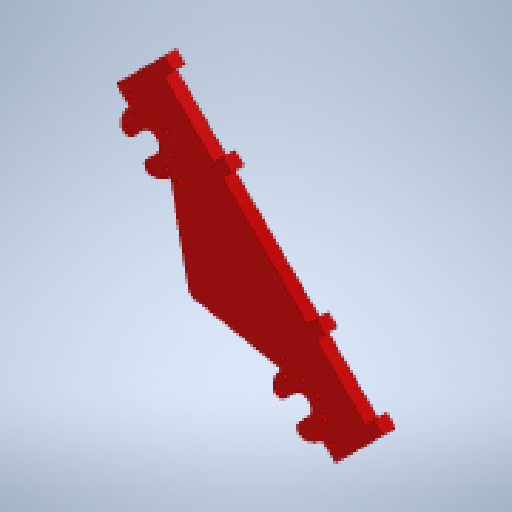
# Autodesk Inventor part: new_waist
Saved by Autodesk Inventor 2024 (Build 280153000, 153)
## iProperties
Created: 2024-09-05
Part Number: new_waist
Material: PMMA 플라스틱
Document SubType Name: Modeling
Designer: Eungang
Density: 1.188 g/cm^3
Appearance: 빨간색
Author: Eungang
Autodesk Inventor part; units mm, degrees
ref_plane "YZ Plane" through (0, 0, 0) normal (1, 0, 0) x (0, 1, 0)
ref_plane "XZ Plane" through (0, 0, 0) normal (0, 1, 0) x (-1, 0, 0)
ref_plane "XY Plane" through (0, 0, 0) normal (0, 0, 1) x (1, 0, 0)
sketch "스케치1" plane through (0, 0, 0) normal (0, 0, 1) x (1, 0, 0)
  circle A0 centre (0, 0) radius 13.8
  circle A1 centre (0, 0) radius 7.2
  circle A2 centre (0, 11) radius 1.28125
  circle A3 centre (-7.778175, 7.778175) radius 1.28125
  circle A4 centre (-11, 0) radius 1.28125
  circle A5 centre (-7.778175, -7.778175) radius 1.28125
  circle A6 centre (0, -11) radius 1.28125
  circle A7 centre (7.778175, -7.778175) radius 1.28125
  circle A8 centre (11, 0) radius 1.28125
  circle A9 centre (7.778175, 7.778175) radius 1.28125
  circle A10 centre (-7.778175, 7.778175) radius 1.025
  circle A11 centre (0, 11) radius 1.025
  circle A12 centre (7.778175, 7.778175) radius 1.025
  circle A13 centre (11, 0) radius 1.025
  circle A14 centre (7.778175, -7.778175) radius 1.025
  circle A15 centre (0, -11) radius 1.025
  circle A16 centre (-7.778175, -7.778175) radius 1.025
  circle A17 centre (-11, 0) radius 1.025
  line L0 (-10.976681, 17.449012) -> (-42.26846, -13.842767)
  line L1 (-9.758074, 9.758074) -> (-14.212846, 14.212846)
  circle A18 centre (0, 0) radius 14
  circle A19 centre (0, 0) radius 4.75
  circle A20 centre (0, 0) radius 4.75
  line L2 (-11, 0) -> (-7.778175, -7.778175)
  line L3 (-7.778175, -7.778175) -> (0, -11)
  arc A21 (10.822466, -8.881116) -> (-13.982149, 0.706764) centre (0, 0) ccw
  circle A22 centre (0, 0) radius 7.2
  line L4 (-3.358757, 3.358757) -> (-7.184819, -0.467305)
  line L5 (3.358757, -3.358757) -> (-0.467305, -7.184819)
  arc A23 (-0.677, -7.168101) -> (-0.467305, -7.184819) centre (0, 0) ccw
  arc A24 (-7.184819, -0.467305) -> (-7.168101, -0.677) centre (0, 0) ccw
  arc A25 (-2.755321, -6.651933) -> (-0.467305, -7.184819) centre (0, 0) ccw
  line L6 (-7.184819, -0.467305) -> (-8.42996, -1.712446)
  line L7 (-0.467305, -7.184819) -> (-1.712446, -8.42996)
  line L8 (-2.287695, -11.943731) -> (-2.434135, -11.509038)
  line L9 (-11.943731, -2.287695) -> (-11.509038, -2.434135)
  arc A26 (-1.712446, -8.42996) -> (-2.434135, -11.509038) centre (0.408874, -10.551281) ccw
  arc A27 (-11.509038, -2.434135) -> (-8.42996, -1.712446) centre (-10.551281, 0.408874) ccw
  arc A28 (-13.982149, 0.706764) -> (-11.943731, -2.287695) centre (-10.985974, 0.555314) ccw
  arc A29 (-2.287695, -11.943731) -> (0.706764, -13.982149) centre (0.555314, -10.985974) ccw
  line L10 (127.899091, -121.42676) -> (96.607312, -152.718539)
  arc A30 (98.085128, -103.723147) -> (114.633788, -123.94404) centre (110.253092, -110.647067) ccw
  circle A31 centre (110.450079, -110.450079) radius 13.8
  circle A32 centre (110.450079, -110.450079) radius 7.2
  circle A33 centre (121.450079, -110.450079) radius 1.28125
  circle A34 centre (118.228254, -118.228254) radius 1.28125
  circle A35 centre (110.450079, -121.450079) radius 1.28125
  circle A36 centre (102.671905, -118.228254) radius 1.28125
  circle A37 centre (99.450079, -110.450079) radius 1.28125
  circle A38 centre (102.671905, -102.671905) radius 1.28125
  circle A39 centre (110.450079, -99.450079) radius 1.28125
  circle A40 centre (118.228254, -102.671905) radius 1.28125
  circle A41 centre (110.450079, -110.450079) radius 14
  line L11 (-25.173001, -46.386205) -> (-26.233662, -45.325545)
  line L12 (-25.173001, -46.386205) -> (-23.758788, -47.800418)
  line L13 (-16.263456, -47.376154) -> (-19.79899, -43.84062)
  line L14 (0, 0) -> (-14.212846, 14.212846)
  line L15 (-16.263456, -47.376154) -> (23.405234, -87.044845)
  line L16 (23.405234, -87.044845) -> (43.23958, -106.87919)
  line L17 (90.988117, -84.515786) -> (59.696338, -115.807565)
  line L18 (-7.656957, -21.021289) -> (-4.793182, -23.885065)
  line L19 (10.20203, -11.383484) -> (18.603693, -52.595148)
  circle A42 centre (73.539105, -73.539105) radius 13.8
  circle A43 centre (73.539105, -73.539105) radius 7.2
  circle A44 centre (84.539105, -73.539105) radius 1.28125
  circle A45 centre (81.31728, -81.31728) radius 1.28125
  circle A46 centre (73.539105, -84.539105) radius 1.28125
  circle A47 centre (65.760931, -81.31728) radius 1.28125
  circle A48 centre (62.539105, -73.539105) radius 1.28125
  circle A49 centre (65.760931, -65.760931) radius 1.28125
  circle A50 centre (73.539105, -62.539105) radius 1.28125
  circle A51 centre (81.31728, -65.760931) radius 1.28125
  circle A52 centre (81.31728, -81.31728) radius 1.025
  circle A53 centre (84.539105, -73.539105) radius 1.025
  circle A54 centre (81.31728, -65.760931) radius 1.025
  circle A55 centre (73.539105, -62.539105) radius 1.025
  circle A56 centre (65.760931, -65.760931) radius 1.025
  circle A57 centre (62.539105, -73.539105) radius 1.025
  circle A58 centre (65.760931, -81.31728) radius 1.025
  circle A59 centre (73.539105, -84.539105) radius 1.025
  line L20 (83.297179, -83.297179) -> (87.751952, -87.751952)
  circle A60 centre (73.539105, -73.539105) radius 14
  circle A61 centre (73.539105, -73.539105) radius 4.75
  circle A62 centre (73.539105, -73.539105) radius 4.75
  line L21 (73.539105, -84.539105) -> (65.760931, -81.31728)
  line L22 (65.760931, -81.31728) -> (62.539105, -73.539105)
  arc A63 (74.245869, -87.521254) -> (64.657989, -62.716639) centre (73.539105, -73.539105) ccw
  circle A64 centre (73.539105, -73.539105) radius 7.2
  line L23 (76.897862, -76.897862) -> (73.071801, -80.723924)
  line L24 (70.180348, -70.180348) -> (66.354286, -74.00641)
  arc A65 (66.354286, -74.00641) -> (66.371004, -74.216105) centre (73.539105, -73.539105) ccw
  arc A66 (72.862105, -80.707206) -> (73.071801, -80.723924) centre (73.539105, -73.539105) ccw
  arc A67 (66.354286, -74.00641) -> (66.887173, -76.294426) centre (73.539105, -73.539105) ccw
  line L25 (73.071801, -80.723924) -> (71.826659, -81.969066)
  line L26 (66.354286, -74.00641) -> (65.109145, -75.251551)
  line L27 (61.595374, -75.8268) -> (62.030067, -75.97324)
  line L28 (71.251411, -85.482837) -> (71.10497, -85.048143)
  arc A68 (62.030067, -75.97324) -> (65.109145, -75.251551) centre (62.987824, -73.130231) ccw
  arc A69 (71.826659, -81.969066) -> (71.10497, -85.048143) centre (73.94798, -84.090386) ccw
  arc A70 (71.251411, -85.482837) -> (74.245869, -87.521254) centre (74.09442, -84.525079) ccw
  arc A71 (59.556956, -72.832341) -> (61.595374, -75.8268) centre (62.553131, -72.983791) ccw
  line L29 (73.539105, -73.539105) -> (87.751952, -87.751952)
  line L30 (52.517816, -81.196062) -> (49.654041, -78.332287)
  line L31 (62.155621, -63.337075) -> (20.943957, -54.935412)
  line L32 (20.85965, -0.353553) -> (-0.353553, 20.85965)
  line L33 (8.768124, 37.193817) -> (110.732922, -64.770981)
  arc A72 (18.603693, -52.595148) -> (20.943957, -54.935412) centre (21.543229, -51.995876) ccw
  arc A73 (10.822466, -8.881116) -> (10.20203, -11.383484) centre (13.141566, -10.784212) ccw
  arc A74 (62.155621, -63.337075) -> (64.657989, -62.716639) centre (62.754893, -60.397539) ccw
  line L34 (4.525483, 32.951176) -> (8.768124, 28.708535)
  line L35 (8.768124, 28.708535) -> (13.010765, 32.951176)
  line L36 (8.768124, 37.193817) -> (13.010765, 32.951176)
  line L37 (4.525483, 32.951176) -> (8.768124, 37.193817)
  line L38 (28.708535, 8.768124) -> (32.951176, 4.525483)
  line L39 (32.951176, 4.525483) -> (37.193817, 8.768124)
  line L40 (32.951176, 13.010765) -> (37.193817, 8.768124)
  line L41 (28.708535, 8.768124) -> (32.951176, 13.010765)
  line L42 (78.064589, -40.587929) -> (82.307229, -44.83057)
  line L43 (82.307229, -44.83057) -> (86.54987, -40.587929)
  line L44 (82.307229, -36.345289) -> (86.54987, -40.587929)
  line L45 (78.064589, -40.587929) -> (82.307229, -36.345289)
  line L46 (102.247641, -64.770981) -> (106.490281, -69.013622)
  line L47 (106.490281, -69.013622) -> (110.732922, -64.770981)
  line L48 (106.490281, -60.52834) -> (110.732922, -64.770981)
  line L49 (102.247641, -64.770981) -> (106.490281, -60.52834)
  line L50 (8.34386, 37.618081) -> (111.157186, -65.195245)
  line L51 (111.157186, -65.195245) -> (74.051758, -102.300674)
  arc A75 (71.223331, -102.300674) -> (74.051758, -102.300674) centre (72.637544, -100.88646) ccw
  line L52 (71.223331, -102.300674) -> (68.394903, -99.472246)
  line L53 (68.394903, -99.472246) -> (97.01505, -70.852099)
  line L54 (97.01505, -70.852099) -> (76.226111, -50.06316)
  line L55 (76.226111, -50.06316) -> (47.605964, -78.683307)
  line L56 (47.605964, -78.683307) -> (44.777537, -75.85488)
  arc A76 (44.777537, -73.026453) -> (44.777537, -75.85488) centre (46.19175, -74.440666) ccw
  line L57 (44.777537, -73.026453) -> (71.98347, -45.820519)
  line L58 (71.98347, -45.820519) -> (27.718586, -1.555635)
  line L59 (27.718586, -1.555635) -> (0.512652, -28.761568)
  arc A77 (-2.315775, -28.761568) -> (0.512652, -28.761568) centre (-0.901561, -27.347355) ccw
  line L60 (-2.315775, -28.761568) -> (-5.144202, -25.933141)
  line L61 (-5.144202, -25.933141) -> (23.475945, 2.687006)
  line L62 (23.475945, 2.687006) -> (2.687006, 23.475945)
  line L63 (2.687006, 23.475945) -> (-25.933141, -5.144202)
  line L64 (-25.933141, -5.144202) -> (-28.761568, -2.315775)
  arc A78 (-28.761568, 0.512652) -> (-28.761568, -2.315775) centre (-27.347355, -0.901561) ccw
  line L65 (-28.761568, 0.512652) -> (8.34386, 37.618081)
  circle A79 centre (15.061374, -9.40452) radius 1.35
  circle A80 centre (-0.494975, -24.960869) radius 1.35
  circle A81 centre (64.134585, -58.477731) radius 1.35
  circle A82 centre (48.578236, -74.03408) radius 1.35
  circle A83 centre (-24.960869, -0.494975) radius 1.35
  circle A84 centre (-9.40452, 15.061374) radius 1.35
  circle A85 centre (73.04413, -98.499975) radius 1.35
  circle A86 centre (88.60048, -82.943625) radius 1.35
  line L66 (106.914545, -60.952605) -> (86.125606, -40.163665)
  line L67 (8.34386, 37.618081) -> (111.157186, -65.195245)
  line L68 (81.882965, -44.406306) -> (86.125606, -40.163665)
  line L69 (77.640325, -40.163665) -> (81.882965, -35.921024)
  line L70 (29.132799, 8.34386) -> (33.37544, 12.586501)
  line L71 (33.37544, 4.101219) -> (37.618081, 8.34386)
  line L72 (-15.945564, 15.945564) -> (-14.212846, 14.212846)
  line L73 (49.709607, 5.444722) -> (53.810826, 9.545942)
  line L74 (11.313708, 43.84062) -> (19.374726, 51.901638)
  line L75 (11.313708, 43.84062) -> (49.709607, 5.444722)
  line L76 (49.709607, 5.444722) -> (53.810826, 9.545942)
  line L77 (11.313708, 43.84062) -> (19.374726, 51.901638)
  line L78 (11.313708, 43.84062) -> (49.709607, 5.444722)
  line L79 (90.161148, -12.652178) -> (85.925733, -16.887593)
  line L80 (85.925733, -16.887593) -> (124.321632, -55.283491)
  line L81 (124.321632, -55.283491) -> (132.368919, -47.236204)
  line L82 (132.368919, -47.236204) -> (128.267699, -43.134985)
  line L83 (128.267699, -43.134985) -> (124.455826, -46.946857)
  line L84 (100.131353, -22.622384) -> (124.455826, -46.946857)
  line L85 (100.131353, -22.622384) -> (103.943226, -18.810511)
  line L86 (103.943226, -18.810511) -> (99.842007, -14.709292)
  line L87 (99.842007, -14.709292) -> (96.030134, -18.521165)
  line L88 (90.161148, -12.652178) -> (96.030134, -18.521165)
  line L89 (11.313708, 43.84062) -> (-31.802127, 0.724784)
  line L90 (-31.802127, 0.724784) -> (-25.933141, -5.144202)
  line L91 (-14.63711, 14.63711) -> (-16.263456, 16.263456)
  line L92 (6.717514, 39.244426) -> (8.768124, 37.193817)
  line L93 (87.751952, -87.751952) -> (89.802561, -89.802561)
  line L94 (89.802561, -89.802561) -> (124.321632, -55.283491)
  line L95 (110.732922, -64.770981) -> (112.783532, -66.821591)
  line L96 (83.933575, -83.933575) -> (106.914545, -60.952605)
  line L97 (62.155621, -63.337075) -> (63.208202, -64.389656)
  line L98 (10.20203, -11.383484) -> (9.14945, -10.330904)
  line L99 (51.901638, 19.374726) -> (47.800418, 23.475945)
  line L100 (23.475945, 47.800418) -> (19.374726, 51.901638)
  line L101 (19.516147, 43.84062) -> (23.475945, 47.800418)
  line L102 (53.810826, 9.545942) -> (47.94184, 15.414928)
  line L103 (47.94184, 15.414928) -> (51.901638, 19.374726)
  line L104 (47.800418, 23.475945) -> (43.84062, 19.516147)
  line L105 (43.84062, 19.516147) -> (19.516147, 43.84062)
  line L106 (51.901638, 19.374726) -> (47.800418, 23.475945)
  line L107 (23.475945, 47.800418) -> (19.374726, 51.901638)
  line L108 (19.516147, 43.84062) -> (23.475945, 47.800418)
  line L109 (53.810826, 9.545942) -> (47.94184, 15.414928)
  line L110 (47.94184, 15.414928) -> (51.901638, 19.374726)
  line L111 (47.800418, 23.475945) -> (43.84062, 19.516147)
  line L112 (43.84062, 19.516147) -> (19.516147, 43.84062)
  point P0 (0, 0)
  point P1 (-3.028175, -9.745689)
  point P2 (-9.745689, -3.028175)
  point P3 (3.570889, -67.2105)
  point P4 (0.706764, -13.982149)
  point P5 (-13.790586, -0.509652)
  point P6 (9.899495, -9.899495)
  point P7 (19, -54.539105)
  point P8 (73.539105, -73.539105)
  point P9 (63.793416, -76.56728)
  point P10 (70.510931, -83.284794)
  point P11 (63.63961, -63.63961)
  point P12 (-0.509652, -13.790586)
  point P13 (-13.982149, 0.706764)
  point P14 (-9.899495, 9.899495)
  point P15 (9.899495, -9.899495)
  point P16 (83.4386, -83.4386)
  point P17 (10.822466, -8.881116)
  point P18 (83.4386, -83.4386)
  point P19 (74.245869, -87.521254)
  point P20 (88.176216, -88.176216)
  point P21 (63.066524, -64.247978)
  point P22 (9.291127, -10.472581)
  dimension "d5" = 3
  dimension "d6" = 3
  dimension "d10" = 3
  constraints: 72 end point, 50 point on circle, 42 centre point, 28 point on line, 18 tangent, 8 coincident, 5 equal radius, 5 perpendicular, 3 parallel, 1 collinear, 1 midpoint, 6 other
  measures "d5" radius of A26
  measures "d6" radius of A29
  measures "d10" radius of A72
extrude "돌출1" add sketch "스케치1" along normal blind 6 contours A0 A29 L8 A26 L7 A1 L14 A3 | A0 L1 A18 L98 | L14 A3 A1 L6 A27 L9 A28 A0 | A0 A28 A18 L1 | L98 A18 A29 A0 | L1 L63 L32 L61 A73 A18 | L14 A10 A3 | A3 L14 A10 | A18 A73 L61 L98 | L1 L72 L65 L50 L37 L34 L35 L33 L41 L38 L39 L45 L42 L43 L49 L46 L96 L54 L55 A74 L31 L57 L58 L59 L19 A73 L61 L62 L63 | L61 A73 L98 | L63 L62 L61 L32 | L14 L4 A1 | A1 L5 A19 L14 | L72 L91 L89 L92 L65 | L59 L58 L57 L31 A72 L19 | L33 L35 L34 L37 | L33 L70 L38 L41 | A74 L55 L97 | L33 L39 L38 L70 | L55 L54 L53 L20 A60 A74 | A74 A60 L97 L55 | A60 L20 A42 L97 | L97 A42 A71 A60 | L96 L46 L47 L50 L51 L93 L20 L53 | A42 L29 A45 A43 L26 A68 L27 A71 | A60 A70 A42 L20 | L96 L33 L47 L46 | L46 L49 L33 L96 | L33 L68 L42 L45 | A42 A70 L28 A69 L25 A43 L29 A45 | L33 L43 L42 L68 | L51 L95 L94 L93 | L29 A61 L24 A43 | A43 L23 L29 | A2 | A4 | A6 | A7 | A8 | A9
sketch "스케치3" plane through (6.717514, 39.244426, 0) normal (0.7071068, 0.7071068, 0) x (-0.7071068, 0.7071068, 0)
  line L0 (-130.199991, -62.5) -> (-130.199991, -58.1)
  line L1 (-129.199991, -57.1) -> (-124.799991, -57.1)
  line L2 (-123.799991, -58.1) -> (-123.799991, -62.5)
  line L3 (-124.799991, -63.5) -> (-129.199991, -63.5)
  line L4 (-25.200009, -57.1) -> (-20.800009, -57.1)
  line L5 (-19.800009, -58.1) -> (-19.800009, -62.5)
  line L6 (-20.800009, -63.5) -> (-25.200009, -63.5)
  line L7 (-26.200009, -62.5) -> (-26.200009, -58.1)
  line L8 (0, -73.4) -> (0, -1.2)
  line L9 (-7.2, 6) -> (-38.8, 6)
  line L10 (-47.2, 6) -> (-102.8, 6)
  line L11 (-111.2, 6) -> (-142.8, 6)
  line L12 (-150, -1.2) -> (-150, -73.4)
  line L13 (-110, 6) -> (-144, 6)
  line L14 (-144, 6) -> (-144, 0)
  line L15 (-144, 0) -> (-110, 0)
  line L16 (-110, 0) -> (-110, 6)
  line L17 (-46, 6) -> (-104, 6)
  line L18 (-104, 6) -> (-104, 0)
  line L19 (-104, 0) -> (-46, 0)
  line L20 (-46, 0) -> (-46, 6)
  line L21 (-6, 6) -> (-40, 6)
  line L22 (-40, 6) -> (-40, 0)
  line L23 (-40, 0) -> (-6, 0)
  line L24 (-6, 0) -> (-6, 6)
  line L25 (-1, -0.2) -> (-5.2, -0.2)
  line L26 (-6.2, 0.8) -> (-6.2, 5)
  line L27 (-39.8, 5) -> (-39.8, 0.8)
  line L28 (-40.8, -0.2) -> (-45.2, -0.2)
  line L29 (-46.2, 0.8) -> (-46.2, 5)
  line L30 (-103.8, 5) -> (-103.8, 0.8)
  line L31 (-104.8, -0.2) -> (-109.2, -0.2)
  line L32 (-110.2, 0.8) -> (-110.2, 5)
  line L33 (-143.8, 5) -> (-143.8, 0.8)
  line L34 (-144.8, -0.2) -> (-149, -0.2)
  arc A0 (-150, -1.2) -> (-149, -0.2) centre (-150, -0.2) ccw
  arc A1 (-1, -0.2) -> (0, -1.2) centre (0, -0.2) ccw
  arc A2 (-6.2, 0.8) -> (-5.2, -0.2) centre (-6.2, -0.2) ccw
  arc A3 (-7.2, 6) -> (-6.2, 5) centre (-6.2, 6) ccw
  arc A4 (-39.8, 5) -> (-38.8, 6) centre (-39.8, 6) ccw
  arc A5 (-40.8, -0.2) -> (-39.8, 0.8) centre (-39.8, -0.2) ccw
  arc A6 (-46.2, 0.8) -> (-45.2, -0.2) centre (-46.2, -0.2) ccw
  arc A7 (-47.2, 6) -> (-46.2, 5) centre (-46.2, 6) ccw
  arc A8 (-103.8, 5) -> (-102.8, 6) centre (-103.8, 6) ccw
  arc A9 (-104.8, -0.2) -> (-103.8, 0.8) centre (-103.8, -0.2) ccw
  arc A10 (-110.2, 0.8) -> (-109.2, -0.2) centre (-110.2, -0.2) ccw
  arc A11 (-111.2, 6) -> (-110.2, 5) centre (-110.2, 6) ccw
  arc A12 (-143.8, 5) -> (-142.8, 6) centre (-143.8, 6) ccw
  arc A13 (-144.8, -0.2) -> (-143.8, 0.8) centre (-143.8, -0.2) ccw
  arc A14 (-130.199991, -62.5) -> (-129.199991, -63.5) centre (-130.199991, -63.5) ccw
  arc A15 (-129.199991, -57.1) -> (-130.199991, -58.1) centre (-130.199991, -57.1) ccw
  arc A16 (-123.799991, -58.1) -> (-124.799991, -57.1) centre (-123.799991, -57.1) ccw
  arc A17 (-124.799991, -63.5) -> (-123.799991, -62.5) centre (-123.799991, -63.5) ccw
  arc A18 (-26.200009, -62.5) -> (-25.200009, -63.5) centre (-26.200009, -63.5) ccw
  arc A19 (-25.200009, -57.1) -> (-26.200009, -58.1) centre (-26.200009, -57.1) ccw
  arc A20 (-19.800009, -58.1) -> (-20.800009, -57.1) centre (-19.800009, -57.1) ccw
  arc A21 (-20.800009, -63.5) -> (-19.800009, -62.5) centre (-19.800009, -63.5) ccw
  circle A22 centre (-89.5, 3) radius 1.3
  circle A23 centre (-60.5, 3) radius 1.3
  circle A24 centre (-127, 3) radius 1.35
  circle A25 centre (-23, 3) radius 1.35
  line L35 (-150, -73.4) -> (0, -73.4)
  circle A26 centre (-75, -33.8) radius 1.6
  point P0 (-23, 0)
  point P1 (-110.2, 6)
  point P2 (-110.2, 0)
  point P3 (-143.8, 0)
  point P4 (-143.8, 6)
  point P5 (-46.2, 6)
  point P6 (-46.2, 0)
  point P7 (-103.8, 0)
  point P8 (-103.8, 6)
  point P9 (-6.2, 6)
  point P10 (-6.2, 0)
  point P11 (-39.8, 0)
  point P12 (-39.8, 6)
  point P13 (-110.2, 6)
  point P14 (-143.8, 6)
  point P15 (-46.2, 6)
  point P16 (-103.8, 6)
  point P17 (-6.2, 6)
  point P18 (-39.8, 6)
  point P19 (-111.179796, 0)
  point P20 (-111.2, 6)
  point P21 (-142.820204, 0)
  point P22 (-142.8, 6)
  point P23 (-47.179796, 0)
  point P24 (-47.2, 6)
  point P25 (-102.820204, 0)
  point P26 (-102.8, 6)
  point P27 (-7.179796, 0)
  point P28 (-7.2, 6)
  point P29 (-38.820204, 0)
  point P30 (-38.8, 6)
  constraints: 24 end point, 6 parallel, 3 horizontal, 3 perpendicular
extrude "돌출3" cut sketch "스케치3" against normal blind 6 contours A2 L26 A3 L21 L24 L23 | L23 A5 L27 A4 L9 A3 L26 A2 | L23 L22 L21 A4 L27 A5 | A13 L33 A12 L11 A11 L32 A10 L15 | L15 L14 L13 A12 L33 A13 | A10 L32 A11 L13 L16 L15 | A6 L29 A7 L17 L20 L19 | L19 A9 L30 A8 L10 A7 L29 A6 | L19 L18 L17 A8 L30 A9 | A22 | A23 | A24 | A25
sketch "스케치4" plane through (2.474874, 35.001786, 0) normal (0.7071068, 0.7071068, 0) x (0, 0, 1)
  circle A0 centre (3, 89.5) radius 1.3
  circle A1 centre (3, 60.5) radius 1.3
  circle A2 centre (3, 127) radius 1.35
  circle A3 centre (3, 23) radius 1.35
  arc A4 (-1.2, 150) -> (-0.2, 149) centre (-0.2, 150) ccw
  line L0 (-1.2, 150) -> (-73.4, 150)
  line L1 (-73.4, 150) -> (-73.4, 0)
  line L2 (-73.4, 0) -> (-1.2, 0)
  arc A5 (-0.2, 1) -> (-1.2, 0) centre (-0.2, 0) ccw
  line L3 (-0.2, 1) -> (-0.2, 5.2)
  arc A6 (0.8, 6.2) -> (-0.2, 5.2) centre (-0.2, 6.2) ccw
  line L4 (0.8, 6.2) -> (5, 6.2)
  arc A7 (6, 7.2) -> (5, 6.2) centre (6, 6.2) ccw
  line L5 (6, 7.2) -> (6, 38.8)
  arc A8 (5, 39.8) -> (6, 38.8) centre (6, 39.8) ccw
  line L6 (5, 39.8) -> (0.8, 39.8)
  arc A9 (-0.2, 40.8) -> (0.8, 39.8) centre (-0.2, 39.8) ccw
  line L7 (-0.2, 40.8) -> (-0.2, 45.2)
  arc A10 (0.8, 46.2) -> (-0.2, 45.2) centre (-0.2, 46.2) ccw
  line L8 (0.8, 46.2) -> (5, 46.2)
  arc A11 (6, 47.2) -> (5, 46.2) centre (6, 46.2) ccw
  line L9 (6, 47.2) -> (6, 102.8)
  arc A12 (5, 103.8) -> (6, 102.8) centre (6, 103.8) ccw
  line L10 (5, 103.8) -> (0.8, 103.8)
  arc A13 (-0.2, 104.8) -> (0.8, 103.8) centre (-0.2, 103.8) ccw
  line L11 (-0.2, 104.8) -> (-0.2, 109.2)
  arc A14 (0.8, 110.2) -> (-0.2, 109.2) centre (-0.2, 110.2) ccw
  line L12 (0.8, 110.2) -> (5, 110.2)
  arc A15 (6, 111.2) -> (5, 110.2) centre (6, 110.2) ccw
  line L13 (6, 111.2) -> (6, 142.8)
  arc A16 (5, 143.8) -> (6, 142.8) centre (6, 143.8) ccw
  line L14 (5, 143.8) -> (0.8, 143.8)
  arc A17 (-0.2, 144.8) -> (0.8, 143.8) centre (-0.2, 143.8) ccw
  line L15 (-0.2, 144.8) -> (-0.2, 149)
  arc A18 (-62.5, 130.199991) -> (-63.5, 129.199991) centre (-63.5, 130.199991) ccw
  line L16 (-62.5, 130.199991) -> (-58.1, 130.199991)
  arc A19 (-57.1, 129.199991) -> (-58.1, 130.199991) centre (-57.1, 130.199991) ccw
  line L17 (-57.1, 129.199991) -> (-57.1, 124.799991)
  arc A20 (-58.1, 123.799991) -> (-57.1, 124.799991) centre (-57.1, 123.799991) ccw
  line L18 (-58.1, 123.799991) -> (-62.5, 123.799991)
  arc A21 (-63.5, 124.799991) -> (-62.5, 123.799991) centre (-63.5, 123.799991) ccw
  line L19 (-63.5, 124.799991) -> (-63.5, 129.199991)
  arc A22 (-62.5, 26.200009) -> (-63.5, 25.200009) centre (-63.5, 26.200009) ccw
  line L20 (-62.5, 26.200009) -> (-58.1, 26.200009)
  arc A23 (-57.1, 25.200009) -> (-58.1, 26.200009) centre (-57.1, 26.200009) ccw
  line L21 (-57.1, 25.200009) -> (-57.1, 20.800009)
  arc A24 (-58.1, 19.800009) -> (-57.1, 20.800009) centre (-57.1, 19.800009) ccw
  line L22 (-58.1, 19.800009) -> (-62.5, 19.800009)
  arc A25 (-63.5, 20.800009) -> (-62.5, 19.800009) centre (-63.5, 19.800009) ccw
  line L23 (-63.5, 20.800009) -> (-63.5, 25.200009)
  circle A26 centre (-33.8, 75) radius 1.6
  point P0 (0, 23)
extrude "돌출4" cut sketch "스케치4" against normal blind 6 contours A0 | A1 | A2 | A3
sketch "스케치5" plane through (0, 0, 6) normal (0, 0, 1) x (1, 0, 0)
  line L0 (22.026376, 23.935565) -> (17.783736, 19.692924)
  line L1 (23.935565, 22.026376) -> (19.692924, 17.783735)
  line L2 (17.783736, 19.692924) -> (19.692924, 17.783735)
  line L3 (17.783736, 19.692924) -> (19.692924, 17.783735)
  line L4 (19.692924, 17.783735) -> (18.73833, 18.73833)
  line L5 (18.73833, 18.73833) -> (16.617009, 16.617009)
  line L6 (16.617009, 16.617009) -> (19.091883, 14.142136)
  line L7 (16.617009, 16.617009) -> (14.142136, 19.091883)
  line L8 (14.142136, 19.091883) -> (12.020815, 16.970563)
  line L9 (12.020815, 16.970563) -> (17.012515, 12.037886)
  line L10 (17.012515, 12.037886) -> (19.091883, 14.142136)
  line L11 (80.25662, -42.77996) -> (84.49926, -38.53732)
  line L12 (84.49926, -38.53732) -> (80.25662, -34.294679)
  line L13 (80.25662, -34.294679) -> (76.013979, -38.53732)
  line L14 (76.013979, -38.53732) -> (35.001786, 2.474874)
  line L15 (35.001786, 2.474874) -> (39.244426, 6.717514)
  line L16 (39.244426, 6.717514) -> (35.001786, 10.960155)
  line L17 (35.001786, 10.960155) -> (30.759145, 6.717514)
  line L18 (30.759145, 6.717514) -> (6.717514, 30.759145)
  line L19 (6.717514, 30.759145) -> (10.960155, 35.001786)
  line L20 (10.960155, 35.001786) -> (6.717514, 39.244426)
  line L21 (6.717514, 39.244426) -> (-16.263456, 16.263456)
  line L22 (-16.263456, 16.263456) -> (-9.899495, 9.899495)
  arc A0 (-9.899495, 9.899495) -> (-13.982149, 0.706764) centre (0, 0) ccw
  arc A1 (-13.982149, 0.706764) -> (-11.943731, -2.287695) centre (-10.985974, 0.555314) ccw
  line L23 (-11.943731, -2.287695) -> (-11.509038, -2.434135)
  arc A2 (-11.509038, -2.434135) -> (-8.42996, -1.712446) centre (-10.551281, 0.408874) ccw
  line L24 (-8.42996, -1.712446) -> (-3.358757, 3.358757)
  arc A3 (3.358757, -3.358757) -> (-3.358757, 3.358757) centre (0, 0) ccw
  line L25 (3.358757, -3.358757) -> (-1.712446, -8.42996)
  arc A4 (-1.712446, -8.42996) -> (-2.434135, -11.509038) centre (0.408874, -10.551281) ccw
  line L26 (-2.434135, -11.509038) -> (-2.287695, -11.943731)
  arc A5 (-2.287695, -11.943731) -> (0.706764, -13.982149) centre (0.555314, -10.985974) ccw
  arc A6 (0.706764, -13.982149) -> (9.291127, -10.472581) centre (0, 0) ccw
  line L27 (9.291127, -10.472581) -> (10.20203, -11.383484)
  line L28 (10.20203, -11.383484) -> (18.603693, -52.595148)
  arc A7 (18.603693, -52.595148) -> (20.943957, -54.935412) centre (21.543229, -51.995876) ccw
  line L29 (20.943957, -54.935412) -> (62.155621, -63.337075)
  line L30 (62.155621, -63.337075) -> (63.066524, -64.247978)
  arc A8 (63.066524, -64.247978) -> (59.556956, -72.832341) centre (73.539105, -73.539105) ccw
  arc A9 (59.556956, -72.832341) -> (61.595374, -75.8268) centre (62.553131, -72.983791) ccw
  line L31 (61.595374, -75.8268) -> (62.030067, -75.97324)
  arc A10 (62.030067, -75.97324) -> (65.109145, -75.251551) centre (62.987824, -73.130231) ccw
  line L32 (65.109145, -75.251551) -> (70.180348, -70.180348)
  arc A11 (76.897862, -76.897862) -> (70.180348, -70.180348) centre (73.539105, -73.539105) ccw
  line L33 (76.897862, -76.897862) -> (71.826659, -81.969066)
  arc A12 (71.826659, -81.969066) -> (71.10497, -85.048143) centre (73.94798, -84.090386) ccw
  line L34 (71.10497, -85.048143) -> (71.251411, -85.482837)
  arc A13 (71.251411, -85.482837) -> (74.245869, -87.521254) centre (74.09442, -84.525079) ccw
  arc A14 (74.245869, -87.521254) -> (83.4386, -83.4386) centre (73.539105, -73.539105) ccw
  line L35 (83.4386, -83.4386) -> (89.802561, -89.802561)
  line L36 (89.802561, -89.802561) -> (112.783532, -66.821591)
  line L37 (112.783532, -66.821591) -> (108.540891, -62.57895)
  line L38 (108.540891, -62.57895) -> (104.29825, -66.821591)
  line L39 (104.29825, -66.821591) -> (80.25662, -42.77996)
  circle A15 centre (7.778175, 7.778175) radius 1.025
  circle A16 centre (11, 0) radius 1.025
  circle A17 centre (7.778175, -7.778175) radius 1.025
  circle A18 centre (0, 11) radius 1.025
  circle A19 centre (-11, 0) radius 1.025
  circle A20 centre (-7.778175, 7.778175) radius 1.025
  circle A21 centre (0, -11) radius 1.025
  circle A22 centre (15.061374, -9.40452) radius 1.35
  circle A23 centre (64.134585, -58.477731) radius 1.35
  circle A24 centre (-9.40452, 15.061374) radius 1.35
  circle A25 centre (88.60048, -82.943625) radius 1.35
  circle A26 centre (73.539105, -84.539105) radius 1.28125
  circle A27 centre (62.539105, -73.539105) radius 1.28125
  circle A28 centre (81.31728, -81.31728) radius 1.28125
  circle A29 centre (81.31728, -65.760931) radius 1.28125
  circle A30 centre (84.539105, -73.539105) radius 1.28125
  circle A31 centre (65.760931, -65.760931) radius 1.28125
  circle A32 centre (73.539105, -62.539105) radius 1.28125
  line L40 (55.507882, -18.031223) -> (59.750523, -13.788582)
  line L41 (90.156115, -56.922096) -> (87.681241, -54.447222)
  line L42 (90.156115, -56.922096) -> (92.630988, -59.39697)
  line L43 (92.630988, -59.39697) -> (90.509668, -61.51829)
  line L44 (90.509668, -61.51829) -> (85.576991, -56.526591)
  line L45 (85.576991, -56.526591) -> (87.681241, -54.447222)
  point P0 (0, 0)
  dimension "d17" = 3
  dimension "d18" = 3.5
  dimension "d19" = 3.5
  dimension "d20" = 3
  constraints: 32 end point, 5 symmetric about line, 3 perpendicular, 2 midpoint, 1 collinear, 6 other
  measures "d17" distance of L4.end L5.end
  measures "d18" distance of L5.end L6.end
  measures "d19" distance of L5.end L7.end
  measures "d20" distance of L7.end L8.end
extrude "돌출5" cut sketch "스케치5" against normal up to next contours L6 L10 L9 L8 L7 | L42 L43 L44 L45 L41
